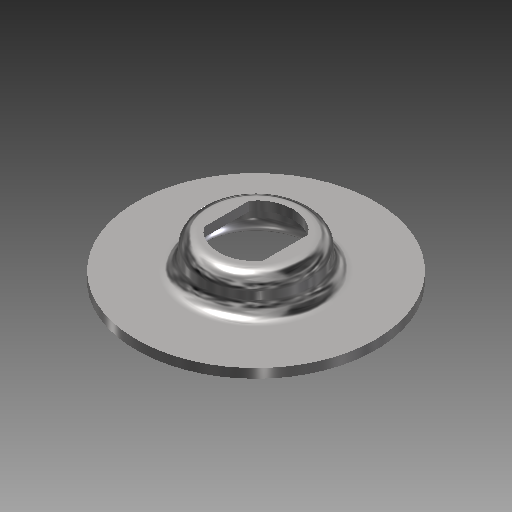
# Autodesk Inventor part: 404-08
Saved by Autodesk Inventor 2019 (Build 230136000, 136)
## iProperties
Company: Autodesk Inc.
Created: 2017-06-27
Part Number: 404-08
Material: Steel, Mild
Document SubType Name: Sheet Metal
Designer: Autodesk Inc.
Mass: 4.48694 g
Surface Area: 12.4954 cm^2
Volume: 0.571584 cm^3
Density: 7.85 g/cm^3
Sheet Metal Rule: Default_mm
Appearance: Semi-Polished
Author: Inventor
Autodesk Inventor part; units mm, degrees
note: some values were not read from the file. Chosen so that the rebuilt part matches the saved one: side of "Thicken2".
ref_plane "YZ Plane" through (0, 0, 0) normal (1, 0, 0) x (0, 1, 0)
ref_plane "XZ Plane" through (0, 0, 0) normal (0, 1, 0) x (-1, 0, 0)
ref_plane "XY Plane" through (0, 0, 0) normal (0, 0, 1) x (1, 0, 0)
sketch "Sketch1" plane through (0, 0, 0) normal (0, 0, 1) x (1, 0, 0)
  line L0 (0, 0) -> (4.5, 0)
  line L1 (6, 0) -> (6, -2.25) construction
  line L2 (7.5, -3.75) -> (13, -3.75)
  line L3 (0, 0) -> (0, 5.6294)
  arc A0 (6, -2.25) -> (7.5, -3.75) centre (7.5, -2.25) ccw
  arc A1 (6, -1.5) -> (4.5, 0) centre (4.5, -1.5) ccw
  line L4 (6, -2.25) -> (6, -1.5)
  point P0 (6, -3.75)
  dimension "d0" = 12
  dimension "d1" = 26
  dimension "d2" = 3.75
  dimension "d3" = 1.5
  constraints: 10 end point, 5 point on circle, 5 tangent, 4 point on line, 2 centre point, 2 perpendicular, 1 collinear, 1 equal radius, 1 horizontal, 1 parallel
  measures "d0" diameter of L1 L3
  measures "d1" diameter of L2.end L3
  measures "d2" distance of L1.start point (6, -3.75)
  measures "d3" radius of A0
surface revolve "RevolutionSrf1" sketch "Sketch1" angle 360 about axis through (0, 0, 0) along (0, 1, 0) shown no curves L2 A0 L4 A1 L0 L3
thicken "Thicken2" operation add thickness 1 both sides no extend neighbours no toward (0, -1, 0) faces at (0.8521, 0, 1.2345) (5.9182, -1.3879, 0.9618) (5.9805, -2, 0.4828) (7.2922, -3.7458, 1.1851) (11.0407, -3.75, 1.037)
sketch "Sketch3" plane through (0, 0, 0) normal (0, 1, 0) x (1, 0, 0)
  circle A0 centre (0, 0) radius 4.05
  line L0 (-3.2, 2.4824) -> (-3.2, -2.4824)
  line L1 (3.2, 2.4824) -> (3.2, -2.4824)
  dimension "d16" = 8.1
  dimension "d17" = 6.4
  constraints: 4 end point, 4 point on circle, 2 parallel, 1 centre point, 1 coincident, 1 vertical
  measures "d16" diameter of A0
  measures "d17" distance between parallel lines of L1 L0
extrude "Extrusion2" cut sketch "Sketch3" against normal through all contours L1 A0 L0
equation "\"BendRadius\" = Thickness"
equation "\"BendReliefWidth\" = Thickness"
equation "\"BendReliefDepth\" = 0.5 * Thickness"
equation "\"CornerReliefSize\" = 4 * Thickness"
equation "\"MinimumRemnant\" = 2 * Thickness"
equation "\"TransitionRadius\" = BendRadius"
equation "\"JacobiRadiusSize\" = BendRadius"
equation "\"Thickness\" = 1"
body "Solid2"
body "Srf1"
